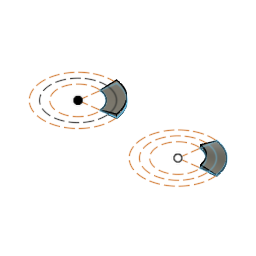
Big Gear Flaps v2 (Autodesk Fusion 360 design; units mm, degrees)
Autodesk Fusion 360 part; units mm, degrees
sketch "Sketch1" plane through (0, 0, 0) normal (0, 1, 0) x (1, 0, 0)
  line L0 (9.0576, 69.3611) -> (15.6355, 119.7334)
  line L1 (69.342, 9.203) -> (119.7004, 15.8865)
  arc A0 (69.342, 9.203) -> (9.0576, 69.3611) centre (0, 0) ccw
  arc A1 (9.0576, 69.3611) -> (69.342, 9.203) centre (0, 0) ccw construction
  arc A2 (94.5212, 12.5448) -> (12.3466, 94.5473) centre (0, 0) ccw
  arc A3 (12.3466, 94.5473) -> (94.5212, 12.5448) centre (0, 0) ccw construction
  arc A4 (119.7004, 15.8865) -> (15.6355, 119.7334) centre (0, 0) ccw
  arc A5 (15.6355, 119.7334) -> (119.7004, 15.8865) centre (0, 0) ccw construction
  line L2 (0, 0) -> (9.0576, 69.3611) construction
  line L3 (0, 0) -> (69.342, 9.203) construction
  line L4 (419.342, 9.203) -> (469.7004, 15.8865)
  arc A6 (419.342, 9.203) -> (359.0576, 69.3611) centre (350, 0) ccw
  arc A7 (362.3466, 94.5473) -> (444.5212, 12.5448) centre (350, 0) ccw construction
  line L5 (350, 0) -> (419.342, 9.203) construction
  arc A8 (444.5212, 12.5448) -> (362.3466, 94.5473) centre (350, 0) ccw
  arc A9 (365.6355, 119.7334) -> (469.7004, 15.8865) centre (350, 0) ccw construction
  arc A10 (359.0576, 69.3611) -> (419.342, 9.203) centre (350, 0) ccw construction
  line L6 (359.0576, 69.3611) -> (365.6355, 119.7334)
  line L7 (350, 0) -> (359.0576, 69.3611) construction
  arc A11 (469.7004, 15.8865) -> (365.6355, 119.7334) centre (350, 0) ccw
  dimension "d1" = 190.7
  dimension "d4" = 75
  dimension "d11" = 190.7
  dimension "d12" = 75
  constraint coincident A0.centre A1.centre
  constraint concentric A0 A2
  constraint concentric A0 A1
  constraint coincident L0 A2.end
  constraint coincident L1 A2.start
  constraint concentric A2 A3
  constraint concentric A4 A5
  constraint coincident A2.end L2
  constraint coincident A2.start L3
  constraint concentric A6 A8
  constraint concentric A6 A10
  constraint coincident A7.start L6
  constraint coincident A7.end L4
  constraint concentric A7 A8
  constraint concentric A9 A11
  constraint coincident A7.start L7
  constraint coincident A7.end L5
  measures "d1" diameter of A2
  measures "d4" angle of L0 L1
  measures "d11" diameter of A8
  measures "d12" angle of L4 L6
extrude "Extrude1" add sketch "Sketch1" along normal blind 10 contours L0 L1 A0 A2 | L0 L1 A2 A4 makes body 1
extrude "Extrude2" add sketch "Sketch1" against normal blind 2.5 contours L0 L1 A2 A4 bodies 1
chamfer "Chamfer1" distance 50 distance2 9 1 edges at (49.4102, 10, -49.5139) measured on face at (84.0019, 10, -60.5603) on bodies 1
extrude "Extrude3" add sketch "Sketch1" along normal blind 10 separate body contours L4 A6 A8 L6 | L4 A8 L6 A11 makes body 2
extrude "Extrude4" add sketch "Sketch1" against normal blind 2.5 contours L4 A8 L6 A11 bodies 2
chamfer "Chamfer2" distance 50 distance2 10 1 edges at (435.2936, 10, -85.4726) measured on face at (434.0019, 10, -60.5603) on bodies 2
